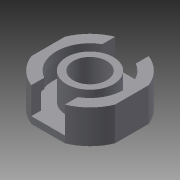
# Autodesk Inventor part: move female
Saved by Autodesk Inventor 2015 (Build 190159000, 159)
## iProperties
Created: 2018-12-22
Part Number: move female
Material: Типовые
Document SubType Name: Modeling
Designer: kostya
Density: 1 g/cm^3
Appearance: По умолчанию
Author: kostya
Autodesk Inventor part; units mm, degrees
ref_plane "YZ Plane" through (0, 0, 0) normal (1, 0, 0) x (0, 1, 0)
ref_plane "XZ Plane" through (0, 0, 0) normal (0, 1, 0) x (-1, 0, 0)
ref_plane "XY Plane" through (0, 0, 0) normal (0, 0, 1) x (1, 0, 0)
sketch "Эскиз7" plane through (0, 0, 0) normal (0, 0, 1) x (1, 0, 0)
  line L0 (-12.5, -12.5) -> (12.5, -12.5)
  line L1 (12.5, -12.5) -> (12.5, 12.5)
  line L2 (12.5, 12.5) -> (-12.5, 12.5)
  line L3 (-12.5, 12.5) -> (-12.5, -12.5)
  line L4 (-12.5, -12.5) -> (12.5, 12.5) construction
  line L5 (12.5, -12.5) -> (-12.5, 12.5) construction
  point P0 (0, 0)
  dimension "d28" = 25
  dimension "d29" = 25
  constraints: 12 end point, 2 midpoint, 2 parallel, 1 horizontal, 1 perpendicular
  measures "d28" distance of L2.end L1.end
  measures "d29" distance of L1.end L0.end
extrude "Выдавливание7" add sketch "Эскиз7" against normal blind 10
sketch "Эскиз8" plane through (0, 0, 0) normal (0, 0, 1) x (1, 0, 0)
  circle A0 centre (0, 0) radius 7
  line L0 (5, 8.6603) -> (5, 10)
  line L1 (-5, 10) -> (-5, 8.6603)
  line L2 (-12.5, -12.5) -> (12.5, -12.5) projected
  line L3 (5, -12.5) -> (-5, -12.5)
  arc A1 (5, -8.6603) -> (5, 8.6603) centre (0, 0) ccw
  arc A2 (-5, 8.6603) -> (-5, -8.6603) centre (0, 0) ccw
  line L4 (-5, -12.5) -> (-5, -8.6603)
  line L5 (-5, 8.6603) -> (-5, 10)
  line L6 (5, 10) -> (5, 8.6603)
  line L7 (5, -8.6603) -> (5, -12.5)
  line L8 (-12.5, 12.5) -> (-12.5, -12.5) construction
  line L9 (-12.5, 0) -> (-7, 0) construction
  line L10 (-5, 10) -> (-5, 12.5)
  line L11 (-5, 12.5) -> (5, 12.5)
  line L12 (12.5, 12.5) -> (-12.5, 12.5) projected
  line L13 (5, 10) -> (5, 12.5)
  dimension "d33" = 14
  dimension "d39" = 5.5
  constraints: 22 end point, 5 parallel, 4 point on circle, 2 centre point, 2 coincident, 2 perpendicular, 2 point on line, 1 horizontal alignment, 1 midpoint, 1 vertical, 2 other
  measures "d39" distance of L9.start L9.end
extrude "Выдавливание8" cut sketch "Эскиз8" against normal blind 8
sketch "Эскиз9" plane through (-5, -12.5, 0) normal (1, 0, 0) x (0, 0, -1)
  line L0 (0, 0) -> (0, 3.8397) projected
  line L1 (8, 0) -> (0, 0) projected
  line L2 (8, 0) -> (8, 3.8397) projected
  line L3 (0, 3.8397) -> (8, 3.8397) projected
  line L4 (0, 0) -> (3, 0) construction
  line L5 (8, 0) -> (0, 0) construction
  line L6 (8, 3.8397) -> (3, 3.8397)
  line L7 (3, 3.8397) -> (3, 2.8397)
  line L8 (3, 2.8397) -> (8, 2.8397)
  line L9 (8, 2.8397) -> (8, 3.8397)
  point P0 (0, 12.5)
  dimension "d38" = 3
  dimension "d40" = 1
  constraints: 10 end point, 2 parallel, 1 horizontal, 1 perpendicular, 1 point on line
  measures "d38" distance of L0.start L4.end
  measures "d40" distance of L7.end L6.end
sketch "Эскиз10" plane through (0, 0, 0) normal (0, 0, 1) x (1, 0, 0)
  line L0 (-4.9924, -8.6432) -> (-5, -9.1432)
  line L1 (-5, -12.5) -> (-5, -8.6603) projected
  circle A0 centre (0, 0) radius 10.421
  dimension "d41" = 0.5
  constraints: 2 end point, 1 coincident, 1 point on line, 3 other
  measures "d41" distance of L0.start L0.end
sweep "Сдвиг1" cut profiles "Эскиз9" path "Эскиз10" path curves A0 contours L3 L2 L8 L7
sketch "Эскиз11" plane through (0, 0, 0) normal (0, 0, 1) x (1, 0, 0)
  circle A0 centre (0, 0) radius 5
  dimension "d44" = 10
  constraints: 1 centre point, 1 coincident
  measures "d44" diameter of A0
extrude "Выдавливание9" cut sketch "Эскиз11" against normal up to surface (10 mm away)
sketch "Эскиз13" plane through (0, 0, 0) normal (0, 0, 1) x (1, 0, 0)
  line L0 (-12.5, 12.5) -> (-5, 12.5)
  line L1 (-5, 12.5) -> (-12.5, 12.5) projected
  line L2 (-5, -12.5) -> (-12.5, -12.5)
  line L3 (-12.5, -12.5) -> (-5, -12.5) projected
  arc A0 (-5, 12.5) -> (-12.5, 5) centre (0, 0) ccw
  arc A1 (-12.5, -5) -> (-5, -12.5) centre (0, 0) ccw
  line L4 (-12.5, -12.5) -> (-12.5, -5)
  line L5 (-12.5, 5) -> (-12.5, 12.5)
  line L6 (0, -12.5) -> (0, 12.5) construction
  line L7 (-5, 12.5) -> (5, 12.5) construction
  line L8 (12.5, 12.5) -> (5, 12.5)
  line L9 (5, -12.5) -> (12.5, -12.5)
  arc A2 (12.5, 5) -> (5, 12.5) centre (0, 0) ccw
  arc A3 (5, -12.5) -> (12.5, -5) centre (0, 0) ccw
  line L10 (12.5, -12.5) -> (12.5, -5)
  line L11 (12.5, 5) -> (12.5, 12.5)
  constraints: 18 end point, 8 point on circle, 5 symmetric about line, 4 centre point, 2 collinear, 2 vertical, 1 coincident, 1 midpoint, 2 other
extrude "Выдавливание10" cut sketch "Эскиз13" against normal blind 10
